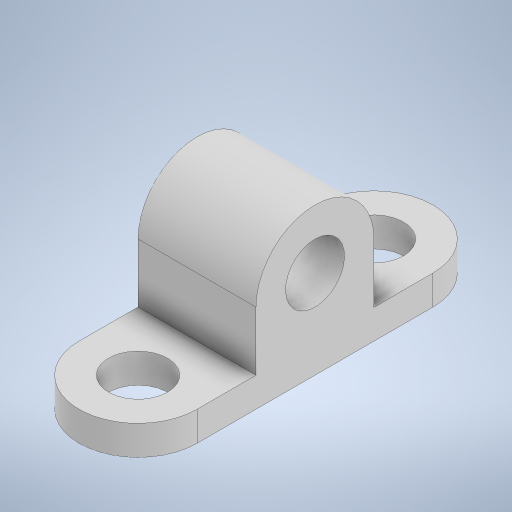
# Autodesk Inventor part: Actividad #1
Saved by Autodesk Inventor 2024.2 (Build 282272000, 272)
## iProperties
Created: 2024-02-04
Part Number: Actividad #1
Material: Generic
Document SubType Name: Modeling
Designer: Josh Juárez
Density: 1 g/cm^3
Appearance: Default
Author: Josh Juárez
Autodesk Inventor part; units mm, degrees
ref_plane "YZ Plane" through (0, 0, 0) normal (1, 0, 0) x (0, 1, 0)
ref_plane "XZ Plane" through (0, 0, 0) normal (0, 1, 0) x (-1, 0, 0)
ref_plane "XY Plane" through (0, 0, 0) normal (0, 0, 1) x (1, 0, 0)
sketch "Sketch1" plane through (0, 0, 0) normal (1, 0, 0) x (0, 1, 0)
  line L0 (0, 0) -> (0, -20)
  line L1 (0, 0) -> (20, 0) construction
  line L2 (0, 0) -> (0, 20)
  line L3 (0, 20) -> (10, 20)
  line L4 (10, 20) -> (10, -20)
  line L5 (10, -20) -> (0, -20)
  line L6 (10, 20) -> (30, 20)
  line L7 (10, -20) -> (30, -20)
  arc A0 (30, -20) -> (30, 20) centre (30, 0) ccw
  circle A1 centre (30, 0) radius 10
  line L8 (10, 20) -> (10, 40)
  line L9 (10, -20) -> (10, -40)
  line L10 (10, -40) -> (0, -40)
  line L11 (0, -40) -> (0, -20)
  line L12 (10, 40) -> (0, 40)
  line L13 (0, 40) -> (0, 20)
  dimension "d0" = 20
  dimension "d1" = 90
  dimension "d2" = 20
  dimension "d3" = 10
  dimension "d4" = 20
  dimension "d5" = 20
  dimension "d7" = 20
  dimension "d8" = 20
  dimension "d9" = 20
  constraints: 28 end point, 5 perpendicular, 4 horizontal, 4 vertical, 2 centre point, 2 point on circle, 2 point on line, 1 coincident, 1 collinear
  measures "d0" distance of L0.start L0.end
  measures "d1" angle of L0 L1
  measures "d2" distance of L0.start L2.end
  measures "d3" distance of L2.end L3.end
  measures "d4" distance of L3.end L6.end
  measures "d5" distance of L7.end L4.end
  measures "d7" diameter of A1
  measures "d8" distance of L3.end L8.end
  measures "d9" distance of L4.end L9.end
extrude "Extrusion1" add sketch "Sketch1" along normal blind 40 contours L2 L3 L4 L5 L0 | L4 L6 A0 L7
sketch "Sketch2" plane through (0, 0, -20) normal (0, 0, -1) x (-1, 0, 0)
  line L0 (-40, 30) -> (-40, 0) projected
  line L1 (-40, 0) -> (0, 0)
  line L2 (0, 0) -> (0, 10)
  line L3 (0, 10) -> (-40, 10)
  dimension "d12" = 10
  constraints: 6 end point, 2 perpendicular, 1 horizontal, 1 point on line
  measures "d12" distance of L1.end L2.end
extrude "Extrusion2" add sketch "Sketch2" along normal blind 20
sketch "Sketch3" plane through (0, 0, 20) normal (0, 0, 1) x (1, 0, 0)
  line L0 (0, 0) -> (40, 0) projected
  line L1 (0, 0) -> (40, 0)
  line L2 (40, 0) -> (40, 10)
  line L3 (40, 10) -> (0, 10)
  line L4 (0, 10) -> (0, 0)
  dimension "d15" = 10
  constraints: 8 end point, 3 perpendicular, 1 collinear
  measures "d15" distance of L0.end L2.end
extrude "Extrusion3" add sketch "Sketch3" along normal blind 20
sketch "Sketch4" plane through (0, 10, 20) normal (0, 1, 0) x (1, 0, 0)
  line L0 (40, -20) -> (0, -20) projected
  circle A0 centre (20, -20) radius 20
  circle A1 centre (20, -20) radius 10
  point P0 (0, 20)
  dimension "d18" = 40
  dimension "d19" = 20
  constraints: 2 centre point, 1 coincident, 1 midpoint
  measures "d18" diameter of A0
  measures "d19" diameter of A1
extrude "Extrusion4" add sketch "Sketch4" against normal blind 10
sketch "Sketch5" plane through (0, 10, 20) normal (0, 1, 0) x (1, 0, 0)
  arc A0 (0, -20) -> (40, -20) centre (20, -20) ccw projected
  circle A1 centre (20, -20) radius 10
  point P0 (0, 20)
  dimension "d22" = 20
  constraints: 1 centre point, 1 coincident
  measures "d22" diameter of A1
extrude "Extrusion5" cut sketch "Sketch5" against normal blind 10
sketch "Sketch6" plane through (0, 10, -20) normal (0, 1, 0) x (1, 0, 0)
  line L0 (40, 20) -> (0, 20) projected
  circle A0 centre (20, 20) radius 20
  circle A1 centre (20, 20) radius 10
  point P0 (0, -20)
  dimension "d25" = 40
  dimension "d26" = 20
  constraints: 2 centre point, 1 coincident, 1 midpoint
  measures "d25" diameter of A0
  measures "d26" diameter of A1
extrude "Extrusion6" add sketch "Sketch6" against normal blind 10
sketch "Sketch7" plane through (0, 10, -20) normal (0, 1, 0) x (1, 0, 0)
  arc A0 (40, 20) -> (0, 20) centre (20, 20) ccw projected
  circle A1 centre (20, 20) radius 10
  point P0 (0, -20)
  dimension "d29" = 20
  constraints: 1 centre point, 1 coincident
  measures "d29" diameter of A1
extrude "Extrusion7" cut sketch "Sketch7" against normal blind 10
body "Solid1"
